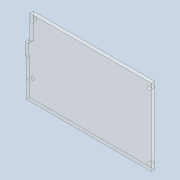
# Autodesk Inventor part: 0008-30-010
Saved by Autodesk Inventor 2020 (Build 240168000, 168)
## iProperties
Created: 2021-05-25
Part Number: 0008-30-010
Material: PET Plastic
Document SubType Name: Modeling
Designer: Iulian Bors
Density: 1.541 g/cm^3
Appearance: Clear
Author: Iulian Bors
Autodesk Inventor part; units mm, degrees
ref_plane "YZ Plane" through (0, 0, 0) normal (1, 0, 0) x (0, 1, 0)
ref_plane "XZ Plane" through (0, 0, 0) normal (0, 1, 0) x (-1, 0, 0)
ref_plane "XY Plane" through (0, 0, 0) normal (0, 0, 1) x (1, 0, 0)
sketch "Sketch1" plane through (0, 0, 0) normal (0, 0, 1) x (1, 0, 0)
  line L0 (-54, 36.5) -> (54, 36.5)
  line L1 (54, 36.5) -> (54, -36.5)
  line L2 (54, -36.5) -> (-54, -36.5)
  line L3 (-54, -36.5) -> (-54, 36.5)
  point P0 (0, 0)
  point P1 (-54, 0)
  point P2 (0, 36.5)
  dimension "d0" = 108
  dimension "d1" = 73
  constraints: 8 end point, 2 midpoint, 2 parallel, 1 horizontal, 1 horizontal alignment, 1 perpendicular, 1 vertical alignment
  measures "d0" distance of L0.start L0.end
  measures "d1" distance of L2.end L0.start
extrude "Extrusion1" add sketch "Sketch1" along normal blind 3
sketch "Sketch2" plane through (0, 0, 0) normal (0, 0, -1) x (-1, 0, 0)
  line L0 (58.5, 13.0157) -> (58.5, 1.0157) projected
  line L1 (57.5, 1.0157) -> (57.5, -42.5) projected
  line L2 (55, 13.0157) -> (58.5, 13.0157) projected
  line L3 (58.5, 1.0157) -> (57.5, 1.0157) projected
  line L4 (58, 12.5157) -> (54, 12.5157)
  line L5 (54, 12.5157) -> (54, 1.5157)
  line L6 (54, 1.5157) -> (58, 1.5157)
  line L7 (58, 1.5157) -> (58, 12.5157)
  line L8 (57, 1.5157) -> (54, 1.5157)
  line L9 (54, 1.5157) -> (54, -36.5)
  line L10 (54, -36.5) -> (57, -36.5)
  line L11 (57, -36.5) -> (57, 1.5157)
  line L12 (54, 36.5) -> (54, -36.5) projected
  line L13 (54, -36.5) -> (-54, -36.5) projected
  point P0 (0, 0)
  point P1 (54, 1.5157)
  dimension "d5" = 0.5
  dimension "d6" = 0.5
  dimension "d7" = 0.5
  dimension "d8" = 0.5
  constraints: 16 end point, 4 parallel, 3 collinear, 2 horizontal, 2 perpendicular, 1 point on line
  measures "d5" distance between parallel lines of L4 L2
  measures "d6" distance between parallel lines of L0 L7
  measures "d7" distance between parallel lines of L3 L6
  measures "d8" distance between parallel lines of L11 L1
extrude "Extrusion2" add sketch "Sketch2" against normal up to surface (3 mm away)
fillet "Fillet1" radius 1.5 2 edges at (-57, 1.5157, 1.5) (-54, 12.5157, 1.5)
sketch "Sketch4" plane through (0, 0, 0) normal (0, 0, -1) x (-1, 0, 0)
  line L0 (57, -31.5) -> (-54, -31.5)
  line L1 (-54, -31.5) -> (-54, -36.5)
  line L2 (-54, -36.5) -> (57, -36.5)
  line L3 (57, -36.5) -> (57, -31.5)
  line L4 (57, -36.5) -> (57, 0.1015) projected
  line L5 (-54, -36.5) -> (57, -36.5) projected
  line L6 (-54, -36.5) -> (-54, 36.5) projected
  line L7 (-54, 36.5) -> (54, 36.5) projected
  point P0 (0, 0)
  dimension "d25" = 68
  constraints: 8 end point, 3 collinear, 2 parallel, 1 horizontal, 1 perpendicular
  measures "d25" distance between parallel lines of L0 L7
extrude "Extrusion3" cut sketch "Sketch4" against normal through all
sketch "Sketch3" plane through (0, 0, 0) normal (0, 0, -1) x (-1, 0, 0)
  circle A0 centre (52, 31.5) radius 1.25 projected
  circle A1 centre (54.5, -15.5) radius 1.25
  circle A2 centre (-52, -26.5) radius 1.25
  circle A3 centre (-52, 31.5) radius 1.25 projected
  line L0 (57, -36.5) -> (57, 1.5157) projected
  line L1 (-54, -36.5) -> (-54, 36.5) projected
  line L2 (-54, -31.5) -> (57, -31.5) projected
  point P0 (0, 0)
  dimension "d19" = 2.5
  dimension "d22" = 2
  dimension "d28" = 16
  dimension "d29" = 5
  constraints: 2 centre point
  measures "d19" distance from line of A1.centre L0
  measures "d22" distance from line of A2.centre L1
  measures "d28" distance from line of A1.centre L2
  measures "d29" distance from line of L2 A2.centre
hole "Hole1" at (52, -26.5, 0) at (52, 31.5, 0) at (-52, 31.5, 0) at (-54.5, -15.5, 0) direction (0, 0, 1) diameter 3 end through all
body "Solid1"
